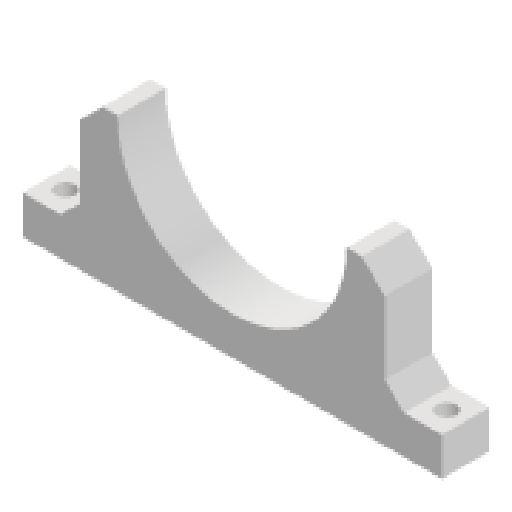
# Autodesk Inventor part: SOPORTE DE GUIA
Saved by Autodesk Inventor 2024 (Build 280153000, 153)
## iProperties
Created: 2024-05-26
Part Number: SOPORTE DE GUIA
Material: Generic
Document SubType Name: Modeling
Designer: Jhuliams
Density: 1 g/cm^3
Appearance: Default
Author: Jhuliams
Autodesk Inventor part; units mm, degrees
ref_plane "YZ Plane" through (0, 0, 0) normal (1, 0, 0) x (0, 1, 0)
ref_plane "XZ Plane" through (0, 0, 0) normal (0, 1, 0) x (-1, 0, 0)
ref_plane "XY Plane" through (0, 0, 0) normal (0, 0, 1) x (1, 0, 0)
sketch "Sketch1" plane through (0, 0, 0) normal (0, 0, 1) x (1, 0, 0)
  line L0 (-80, 80) -> (80, 80)
  line L1 (80, 80) -> (80, -80)
  line L2 (80, -80) -> (-80, -80)
  line L3 (-80, -80) -> (-80, 80)
  line L4 (-80, 80) -> (80, -80) construction
  line L5 (80, 80) -> (-80, -80) construction
  circle A0 centre (0, 0) radius 60
  line L6 (-60, 0) -> (-80, 0)
  line L7 (60, 0) -> (80, 0)
  line L8 (-110, -100) -> (110, -100)
  line L9 (110, -100) -> (110, -60)
  line L10 (110, -60) -> (-110, -60)
  line L11 (-110, -60) -> (-110, -100)
  line L12 (-110, -100) -> (110, -60) construction
  line L13 (110, -100) -> (-110, -60) construction
  point P0 (0, -80)
  point P1 (-80, -60)
  point P2 (80, -60)
  dimension "d0" = 160
  dimension "d1" = 160
  dimension "d2" = 120
  dimension "d5" = 220
  dimension "d6" = 40
  constraints: 28 end point, 7 midpoint, 4 parallel, 2 horizontal, 2 perpendicular, 2 point on circle, 1 centre point, 1 coincident, 1 point on line
  measures "d0" distance of L1.end L2.end
  measures "d1" distance of L0.end L1.end
  measures "d2" diameter of A0
  measures "d5" distance of L10.end L9.end
  measures "d6" distance of L9.end L8.end
extrude "Extrusion1" add sketch "Sketch1" along normal mid plane 25 contours L6 A0 L10 L3 | L1 L10 A0 L7 | L10 L1 L2 L3 | L3 L2 L1 L10 L9 L8 L11
chamfer "Chamfer1" distance 10 angle 45 2 edges at (-80, -60, 0) (80, -60, 0)
sketch "Sketch2" plane through (0, 0, 12.5) normal (0, 0, 1) x (1, 0, 0)
  line L0 (-138.1125, -80) -> (138.1125, -80)
  line L1 (138.1125, -80) -> (138.1125, -120)
  line L2 (138.1125, -120) -> (-138.1125, -120)
  line L3 (-138.1125, -120) -> (-138.1125, -80)
  line L4 (-110, -100) -> (110, -100) projected
  line L5 (-138.1125, -80) -> (138.1125, -120) construction
  line L6 (138.1125, -80) -> (-138.1125, -120) construction
  point P0 (0, 0)
  point P1 (0, -100)
  dimension "d12" = 40
  constraints: 12 end point, 3 midpoint, 2 parallel, 1 horizontal, 1 perpendicular
  measures "d12" distance of L0.end L1.end
extrude "Extrusion2" cut sketch "Sketch2" against normal blind 25
sketch "Sketch3" plane through (-110, -60, 12.5) normal (0, 1, 0) x (1, 0, 0)
  line L0 (20, 25) -> (20, 0) projected
  line L1 (0, 25) -> (20, 25) projected
  line L2 (0, 25) -> (0, 0) projected
  line L3 (20, 0) -> (0, 0) projected
  line L4 (0, 0) -> (20, 25) construction
  line L5 (0, 25) -> (20, 0) construction
  circle A0 centre (10, 12.5) radius 5
  line L6 (110, 12.5) -> (110, 50.8) construction
  circle A1 centre (210, 12.5) radius 5
  dimension "d15" = 10
  constraints: 6 end point, 2 centre point, 1 midpoint, 1 symmetric about line, 1 vertical, 1 other
  measures "d15" diameter of A0
extrude "Extrusion3" cut sketch "Sketch3" against normal blind 25 contours A0 | A1
chamfer "Chamfer2" distance 12 angle 45 1 edges at (80, 0, 0)
chamfer "Chamfer3" distance 12 angle 45 1 edges at (-80, 0, 0)
body "Solid1"
